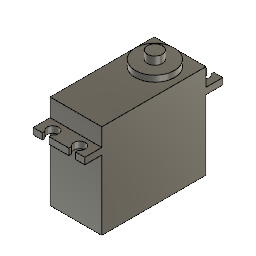
Servo HS-311 _Dim (Autodesk Fusion 360 design; units mm, degrees)
Autodesk Fusion 360 part; units mm, degrees
sketch "Sketch1" plane through (0, 0, 0) normal (0, 0, 1) x (1, 0, 0)
  line L0 (0, 0) -> (19.82, 0)
  line L1 (19.82, 0) -> (19.82, 39.88)
  line L2 (19.82, 39.88) -> (0, 39.88)
  line L3 (0, 39.88) -> (0, 0)
  line L4 (0, 46.36) -> (19.82, 46.36)
  line L5 (19.82, 46.36) -> (19.82, -6.48)
  line L6 (19.82, -6.48) -> (0, -6.48)
  line L7 (0, -6.48) -> (0, 46.36)
  line L8 (9.91, 39.88) -> (9.91, 0) construction
  line L9 (19.82, 19.94) -> (0, 19.94) construction
  circle A0 centre (4.825, 43.57) radius 2.19
  circle A1 centre (14.995, 43.57) radius 2.19
  circle A2 centre (4.825, -3.69) radius 2.19
  circle A3 centre (14.995, -3.69) radius 2.19
  line L10 (3.575, 46.36) -> (3.575, 45.3682)
  line L11 (6.075, 46.36) -> (6.075, 45.3682)
  line L12 (13.745, 46.36) -> (13.745, 45.3682)
  line L13 (16.245, 46.36) -> (16.245, 45.3682)
  line L14 (3.575, -6.48) -> (3.575, -5.4882)
  line L15 (6.075, -6.48) -> (6.075, -5.4882)
  line L16 (13.745, -6.48) -> (13.745, -5.4882)
  line L17 (16.245, -6.48) -> (16.245, -5.4882)
  point P0 (4.825, 43.57)
  point P1 (14.995, 43.57)
  point P2 (4.825, -3.69)
  point P3 (14.995, -3.69)
  dimension "d1" = 19.82
  dimension "d2" = 39.88
  dimension "d3" = 52.84
  dimension "d4" = 47.26
  dimension "d5" = 10.17
  dimension "d15" = 4.38
  dimension "d16" = 2.5
  dimension "d17" = 2.5
  constraint horizontal L0
  constraint vertical L1
  constraint horizontal L2
  constraint vertical L3
  constraint coincident L0.start L3.end
  constraint horizontal L4
  constraint vertical L5
  constraint horizontal L6
  constraint vertical L7
  constraint midpoint L3 L7
  constraint collinear L1 L5
  constraint midpoint L2 L8.start
  constraint midpoint L0 L8.end
  constraint midpoint L1 L9.start
  constraint midpoint L3 L9.end
  constraint symmetric P0 P1 L8
  constraint symmetric P0 L9 P2
  constraint symmetric P1 L9 P3
  constraint coincident P0 A0.centre
  constraint coincident P1 A1.centre
  constraint coincident P2 A2.centre
  constraint coincident P3 A3.centre
  constraint equal A0 A1
  constraint equal A0 A2
  constraint equal A0 A3
  constraint coincident L4 L10.start
  constraint coincident A0 L10.end
  constraint perpendicular L4 L10
  constraint coincident L4 L11.start
  constraint coincident A0 L11.end
  constraint perpendicular L4 L11
  constraint coincident L4 L12.start
  constraint coincident A1 L12.end
  constraint perpendicular L4 L12
  constraint coincident L4 L13.start
  constraint coincident A1 L13.end
  constraint perpendicular L4 L13
  constraint coincident L6 L14.start
  constraint coincident A2 L14.end
  constraint perpendicular L6 L14
  constraint coincident L6 L15.start
  constraint coincident A2 L15.end
  constraint perpendicular L6 L15
  constraint coincident L6 L16.start
  constraint coincident A3 L16.end
  constraint perpendicular L6 L16
  constraint coincident L6 L17.start
  constraint coincident A3 L17.end
  constraint perpendicular L6 L17
  constraint collinear L10 L14
  constraint collinear L11 L15
  constraint collinear L12 L16
  constraint collinear L13 L17
  constraint equal L10 L11
  constraint equal L12 L13
  measures "d1" distance of L0.start L0.end
  measures "d2" distance of L0.start L2.end
  measures "d3" distance of L4.start L6.end
  measures "d4" distance of P1 P3
  measures "d5" distance of P0 P1
  measures "d15" diameter of A0
  measures "d16" distance of L10 L11
  measures "d17" distance of L12 L13
extrude "Extrude1" add sketch "Sketch1" along normal blind 9.35 and the other way blind 26.67 contours L0 L1 L2 L3 L5 L7
extrude "Extrude2" add sketch "Sketch1" along normal blind 2.5 contours L0 L5 L6 L7 A2 A3 L14 L15 L16 L17 | L2 L4 L5 L7 A0 A1 L10 L11 L12 L13
sketch "Sketch3" plane through (0, 0, 9.35) normal (0, 0, 1) x (-1, 0, 0)
  line L0 (-19.82, -39.88) -> (0, -39.88)
  line L1 (0, -39.88) -> (0, 0)
  line L2 (0, 0) -> (-19.82, 0)
  line L3 (-19.82, 0) -> (-19.82, -39.88)
  circle A0 centre (-9.91, -30.22) radius 7.5
  circle A1 centre (-9.91, -30.22) radius 2.88
  line L4 (-9.91, -39.88) -> (-9.91, -30.22) construction
  dimension "d19" = 9.66
  dimension "d20" = 15
  dimension "d21" = 5.76
  constraint concentric A0 A1
  constraint midpoint L0 L4.start
  constraint perpendicular L0 L4
  constraint coincident A0.centre A1.centre
  measures "d19" distance of L4.start A0.centre
  measures "d20" diameter of A0
  measures "d21" diameter of A1
extrude "Extrude3" add sketch "Sketch3" along normal blind 2.33 contours A0
extrude "Extrude4" add sketch "Sketch3" along normal blind 5.38 contours A1
equation "d4 = 13.47 mm + 33.79 mm"
equation "d21 = ( 2.88 * 2 ) * 1 mm"
equation "d22 = 11.68 mm - 9.35 mm"
equation "d24 = 11.68 mm - 9.35 mm + 3.05 mm"
